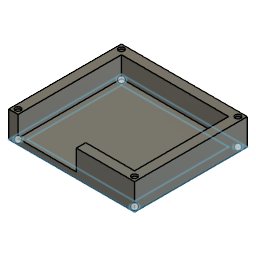
Audiovis (Autodesk Fusion 360 design; units mm, degrees)
part number: 2025-12-09-04-06-24-838
Autodesk Fusion 360 part; units mm, degrees
sketch "Sketch1" plane through (0, 0, 0) normal (0, 1, 0) x (1, 0, 0)
  line L0 (-0.3317, -1.9864) -> (56.6183, -1.9864)
  line L1 (56.6183, -1.9864) -> (56.6183, -51.9564)
  line L2 (56.6183, -51.9564) -> (-0.3317, -51.9564)
  line L3 (-0.3317, -51.9564) -> (-0.3317, -1.9864)
  line L4 (-5.3317, 3.0136) -> (61.6183, 3.0136)
  line L5 (61.6183, 3.0136) -> (61.6183, -56.9564)
  line L6 (61.6183, -56.9564) -> (-5.3317, -56.9564)
  line L7 (-5.3317, -56.9564) -> (-5.3317, 3.0136)
  circle A0 centre (59.1183, -54.4564) radius 1.5
  circle A1 centre (-2.8317, -54.4564) radius 1.5
  circle A2 centre (-2.8317, 0.5136) radius 1.5
  circle A3 centre (59.1183, 0.5136) radius 1.5
  circle A4 centre (-2.8317, -54.4564) radius 2
  circle A5 centre (59.1183, -54.4564) radius 2
  circle A6 centre (59.1183, 0.5136) radius 2
  circle A7 centre (-2.8317, 0.5136) radius 2
  dimension "d2" = 49.97
  dimension "d3" = 66.95
  dimension "d4" = 59.97
  dimension "d5" = 5
  dimension "d6" = 5
  dimension "d7" = 3
  dimension "d8" = 3
  dimension "d9" = 3
  dimension "d10" = 3
  dimension "d11" = 2.5
  dimension "d12" = 2.5
  dimension "d13" = 2.5
  dimension "d14" = 2.5
  dimension "d15" = 2.5
  dimension "d16" = 2.5
  dimension "d17" = 2.5
  dimension "d18" = 2.5
  dimension "d19" = 4
  dimension "d20" = 4
  dimension "d21" = 4
  dimension "d22" = 4
  constraint horizontal L0
  constraint vertical L1
  constraint horizontal L2
  constraint vertical L3
  constraint horizontal L4
  constraint vertical L5
  constraint horizontal L6
  constraint vertical L7
  constraint concentric A1 A4
  constraint concentric A0 A5
  constraint concentric A3 A6
  constraint concentric A2 A7
  measures "d2" distance of L0.start L2.end
  measures "d3" distance of L4.start L4.end
  measures "d4" distance of L4.start L6.end
  measures "d5" distance of L2 L6
  measures "d6" distance of L1 L5
  measures "d7" diameter of A0
  measures "d8" diameter of A1
  measures "d9" diameter of A2
  measures "d10" diameter of A3
  measures "d11" distance of L4 A3.centre
  measures "d12" distance of L5 A3.centre
  measures "d13" distance of L5 A0.centre
  measures "d14" distance of L6 A0.centre
  measures "d15" distance of L6 A1.centre
  measures "d16" distance of L7 A1.centre
  measures "d17" distance of L7 A2.centre
  measures "d18" distance of L4 A2.centre
  measures "d19" diameter of A4
  measures "d20" diameter of A5
  measures "d21" diameter of A6
  measures "d22" diameter of A7
extrude "Extrude1" add sketch "Sketch1" along normal blind 3 contours L0 L1 L2 L3
extrude "Extrude2" add sketch "Sketch1" along normal blind 14 contours L4 L5 L6 L7 | A4 | A5 | A6 | A7
extrude "Extrude3" add sketch "Sketch1" along normal blind 13 contours A0 | A1 | A2 | A3
sketch "Sketch2" plane through (0, 14, 0) normal (0, 1, 0) x (-1, 0, 0)
  circle A0 centre (2.8317, 54.4564) radius 1.5
  circle A1 centre (-59.1183, -0.5136) radius 1.5
  circle A2 centre (-59.1183, 54.4564) radius 1.5
  line L0 (-56.6183, 51.9564) -> (0.3317, 51.9564)
  line L1 (0.3317, 51.9564) -> (0.3317, 1.9864)
  line L2 (0.3317, 1.9864) -> (-56.6183, 1.9864)
  line L3 (-56.6183, 1.9864) -> (-56.6183, 51.9564)
  circle A3 centre (2.8317, -0.5136) radius 1.5
  line L4 (5.3317, 56.9564) -> (-61.6183, 56.9564)
  line L5 (-61.6183, 56.9564) -> (-61.6183, -3.0136)
  line L6 (-61.6183, -3.0136) -> (5.3317, -3.0136)
  line L7 (5.3317, -3.0136) -> (5.3317, 56.9564)
  line L8 (0.3317, 1.9864) -> (-30.6683, 1.9864)
  line L9 (-30.6683, 1.9864) -> (-30.6683, -3.0136)
  line L10 (-30.6683, -3.0136) -> (0.3317, -3.0136)
  line L11 (0.3317, -3.0136) -> (0.3317, 1.9864)
  line L12 (0.3317, 51.9564) -> (-30.6683, 51.9564)
  line L13 (-30.6683, 51.9564) -> (-30.6683, 56.9564)
  line L14 (-30.6683, 56.9564) -> (0.3317, 56.9564)
  line L15 (0.3317, 56.9564) -> (0.3317, 51.9564)
  dimension "d29" = 31
  dimension "d30" = 31
  constraint horizontal L8
  constraint vertical L9
  constraint horizontal L10
  constraint vertical L11
  constraint coincident L6 L9.end
  constraint coincident L1.end L2.start
  constraint horizontal L12
  constraint vertical L13
  constraint horizontal L14
  constraint vertical L15
  constraint coincident L4 L13.end
  constraint coincident L0.end L1.start
  measures "d29" distance of L1.end L8.end
  measures "d30" distance of L0.end L12.end
extrude "Extrude4" cut sketch "Sketch2" against normal blind 11 contours L0 L4 L12 L13 L14 L15
